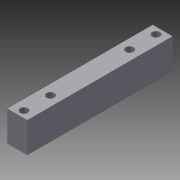
# Autodesk Inventor part: D-042
Saved by Autodesk Inventor 2015 (Build 190159000, 159)
## iProperties
Company: MARCHA TECHNOLOGY
Created: 2013-09-29
Part Number: D-042
Material: Aluminum-6061
Document SubType Name: Modeling
Designer: O.Martin.
Mass: 99.6155 g
Surface Area: 98.9593 cm^2
Volume: 36.7585 cm^3
Density: 2.71 g/cm^3
Project: WITBOXprinter_K01
Description: AMARRE PATIN
Stock Number: 28655
Appearance: Aluminio mate
Author: O.Martin
Autodesk Inventor part; units mm, degrees
ref_plane "YZ Plane" through (0, 0, 0) normal (1, 0, 0) x (0, 1, 0)
ref_plane "XZ Plane" through (0, 0, 0) normal (0, 1, 0) x (-1, 0, 0)
ref_plane "XY Plane" through (0, 0, 0) normal (0, 0, 1) x (1, 0, 0)
sketch "Boceto1" plane through (0, 0, 0) normal (0, 0, 1) x (1, 0, 0)
  line L0 (7.5, -55) -> (-7.5, -55)
  line L1 (-7.5, -55) -> (-7.5, 55)
  line L2 (-7.5, 55) -> (7.5, 55)
  line L3 (7.5, 55) -> (7.5, -55)
  point P0 (0, 0)
  point P1 (0, -55)
  point P2 (7.5, 0)
  dimension "d0" = 15
  dimension "d1" = 110
  constraints: 8 end point, 2 midpoint, 2 parallel, 1 horizontal, 1 horizontal alignment, 1 perpendicular, 1 vertical alignment
  measures "d0" distance of L1.end L2.end
  measures "d1" distance of L0.end L1.end
extrude "Extrusión1" add sketch "Boceto1" against normal blind 23
sketch "Boceto2" plane through (0, 0, 0) normal (0, 0, 1) x (1, 0, 0)
  line L0 (7.5, 55) -> (7.5, -55) projected
  line L1 (-7.5, 55) -> (7.5, 55) projected
  line L2 (0, 50) -> (0, -50) construction
  point P0 (0, 0)
  point P1 (7.5, 0)
  point P2 (0, 55)
  point P3 (0, -30)
  point P4 (0, 30)
  dimension "d4" = 100
  dimension "d5" = 20
  dimension "d6" = 20
  constraints: 3 midpoint, 2 coincident, 2 end point, 2 point on line, 1 horizontal alignment, 1 parallel, 1 vertical alignment
  measures "d4" distance of L2.start L2.end
  measures "d5" distance of point (0, 50) point (0, 30)
  measures "d6" distance of point (0, -50) point (0, -30)
hole "Agujero1" at (0, 50, 0) at (0, -50, 0) at (0, -30, 0) at (0, 30, 0) direction (0, 0, -1) diameter 4.2 end through all counterbore diameter 6 counterbore depth 6
sketch "Boceto3" plane through (0, 0, -23) normal (0, 0, -1) x (-1, 0, 0)
  circle A0 centre (0, 30) radius 2.1 projected
  circle A1 centre (0, -30) radius 2.1 projected
extrude "Extrusión2" add sketch "Boceto3" against normal up to surface (17 mm away)
chamfer "Chaflán1" distance 0.9 angle 31 1 edges at (0, -47.9, -6) measured on face at (0, -47.4, -6)
chamfer "Chaflán2" distance 0.9 angle 31 1 edges at (0, 52.1, -6) measured on face at (0, 52.6, -6)
sketch "Boceto4" plane through (0, -30, -6) normal (0, 0, 1) x (1, 0, 0)
  circle A0 centre (0, 0) radius 3 projected
  circle A1 centre (0, 60) radius 3 projected
  constraints: 2 coincident
hole "Agujero2" at (0, -30, -6) at (0, 30, -6) direction (0, 0, -1) diameter 6 depth 0.01 tip angle 118
equation "\"d6\" = d5"
body "Solid1"
